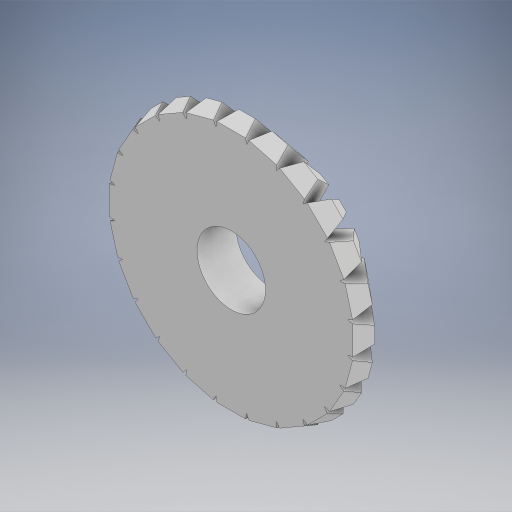
# Autodesk Inventor part: small gear
Saved by Autodesk Inventor 2024 (Build 280153000, 153)
## iProperties
Created: 2024-04-10
Part Number: small gear
Material: Generic
Document SubType Name: Modeling
Designer: Alex
Density: 1 g/cm^3
Appearance: Default
Author: Alex
Autodesk Inventor part; units mm, degrees
sketch "Sketch2" plane through (0, 0, 0) normal (0, 1, 0) x (-1, 0, 0)
  line L0 (0, 0) -> (-24, 0) construction
  line L1 (-24, 0) -> (-16, -8)
  line L2 (-16, -8) -> (-7, -8)
  line L3 (0, 0) -> (0, -8) construction
  line L4 (-7, 0) -> (-7, -8)
  line L5 (-7, -8) -> (0, -8) construction
  line L6 (-24, 0) -> (-7, 0)
  dimension "d3" = 24
  dimension "d4" = 45
  dimension "d5" = 8
  dimension "d6" = 7
  constraints: 14 end point, 3 horizontal, 2 perpendicular, 1 collinear, 1 point on line, 1 vertical
  measures "d3" distance of L0.start L0.end
  measures "d4" angle of L0 L1
  measures "d5" distance between parallel lines of L0 L2
  measures "d6" distance between parallel lines of L3 L4
revolve "Revolution1" add sketch "Sketch2" angle 360 about axis through (0, 0, 0) along (0, 0, -1)
sketch "Sketch3" plane through (0, 0, 0) normal (0, 1, 0) x (-1, 0, 0)
  line L0 (-24, 0) -> (-16, -8) construction
  point P0 (0, 0)
ref_plane "Work Plane6" through (0, 0, 0) normal (0.1323285, 0.9912059, 0) x (0, 0, 1)
ref_plane "Work Plane7" through (0, 0, 0) normal (-0.1323284, 0.9912059, 0) x (0, 0, 1)
sketch "Sketch5" plane through (0, 0, 0) normal (0.1323285, 0.9912059, 0) x (0, 0, 1)
  line L0 (-8, 16) -> (-8, -16) construction
  line L1 (-8, 16) -> (-8, -16) construction
  line L2 (0, 24) -> (0, -24) construction
  line L3 (0, 24) -> (0, -24) construction
  line L4 (-8, -16) -> (0, -24) construction
  line L5 (0, -24) -> (-8, -16) projected
  point P0 (0, 0)
  constraints: 2 end point, 1 collinear
sketch "Sketch6" plane through (0, 0, 0) normal (-0.1323284, 0.9912059, 0) x (0, 0, 1)
  line L0 (-8, 16) -> (-8, -16) projected
  line L1 (0, 24) -> (0, -24) projected
  line L2 (-8, -16) -> (0, -24) construction
  point P0 (0, 0)
  constraints: 2 end point
ref_plane "Work Plane9" through (0, 0, 0) normal (0.703977, 0, -0.7102228) x (0, 1, 0)
ref_plane "Work Plane8" through (-15.8593, 2.1173, -8) normal (0.7102228, 0, 0.703977) x (-0.7008884, 0.0935704, 0.7071068)
sketch "Sketch7" plane through (-15.8593, 2.1173, -8) normal (0.7102228, 0, 0.703977) x (-0.7008884, 0.0935704, 0.7071068)
  line L0 (-0.3962, 4.2159) -> (10.7194, 6.3239) construction
  line L1 (0, 0) -> (11.3137, 0) construction
  line L2 (-0.3962, 4.2159) -> (0, 0) construction
  line L3 (10.7194, 6.3239) -> (11.3137, 0) construction
  point P0 (-5.6569, 1.5949)
  constraints: 4 end point, 1 parallel
ref_plane "Work Plane10" through (-15.8593, 2.1173, -8) normal (0.703977, 0, -0.7102228) x (0, 1, 0)
sketch "Sketch8" plane through (-3.8598, 0, 3.894) normal (0.703977, 0, -0.7102228) x (0, 1, 0)
  line L0 (-2.1173, -16.8954) -> (2.1173, -16.8954) construction
  line L1 (2.1173, -16.8954) -> (-2.1173, -16.8954)
  line L2 (2.1173, -16.8954) -> (1.0253, -19.8954)
  line L3 (1.0253, -19.8954) -> (-1.0253, -19.8954)
  line L4 (-1.0253, -19.8954) -> (-2.1173, -16.8954)
  point P0 (0, 0)
  dimension "d15" = 3
  dimension "d18" = 70
  constraints: 8 end point, 1 collinear, 1 equal length, 1 parallel
  measures "d15" distance between parallel lines of L0 L3
  measures "d18" angle of L0 L4
extrude "Extrusion2" add sketch "Sketch8" along normal up to surface draft 5 surface through (24, 0, 0) normal (0, 0, 1)
chamfer "Chamfer1" distance 5 angle 45 1 edges at (-29.9334, 0, 0)
pattern_circular "Circular Pattern1" count 24 over 360 about axis through (0, 0, -10) along (0, 0, 1) of "Extrusion2", "Chamfer1"
body "Solid2"
